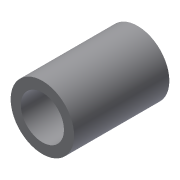
# Autodesk Inventor part: OPENTRONS_Autofocus_clutch_Nema
Saved by Autodesk Inventor 2019.4 (Build 234330000, 330)
## iProperties
Created: 2021-01-06
Part Number: OPENTRONS_Autofocus_clutch_Nema
Material: Generic
Document SubType Name: Modeling
Designer: diederichbenedict
Density: 1 g/cm^3
Appearance: Default
Author: diederichbenedict
Autodesk Inventor part; units mm, degrees
ref_plane "YZ Plane" through (0, 0, 0) normal (1, 0, 0) x (0, 1, 0)
ref_plane "XZ Plane" through (0, 0, 0) normal (0, 1, 0) x (-1, 0, 0)
ref_plane "XY Plane" through (0, 0, 0) normal (0, 0, 1) x (1, 0, 0)
sketch "Sketch1" plane through (0, 0, 0) normal (0, 0, 1) x (1, 0, 0)
  circle A0 centre (0, 0) radius 2.5 projected
  circle A1 centre (0, 0) radius 2.6
  line L0 (-1.3981, 2.1921) -> (1.3981, 2.1921)
  circle A2 centre (0, 0) radius 5
  dimension "d0" = 0.1
  dimension "d1" = 10
  constraints: 2 centre point, 2 end point, 2 point on circle, 1 coincident, 1 horizontal
  measures "d0" radial gap between concentric circles of A0 A1
  measures "d1" diameter of A2
extrude "Extrusion1" add sketch "Sketch1" against normal blind 10
sketch "Sketch2" plane through (0, 0, 0) normal (0, 0, 1) x (1, 0, 0)
  circle A0 centre (0, 0) radius 3.75 projected
  circle A1 centre (0, 0) radius 2.6 projected
  circle A2 centre (0, 0) radius 5 projected
  circle A3 centre (0, 0) radius 1.8
  dimension "d4" = 3.6
  constraints: 1 centre point, 1 coincident
  measures "d4" diameter of A3
extrude "Extrusion2" add sketch "Sketch2" along normal blind 3.6 contours A0 | A1 | A2
body "Solid1"
